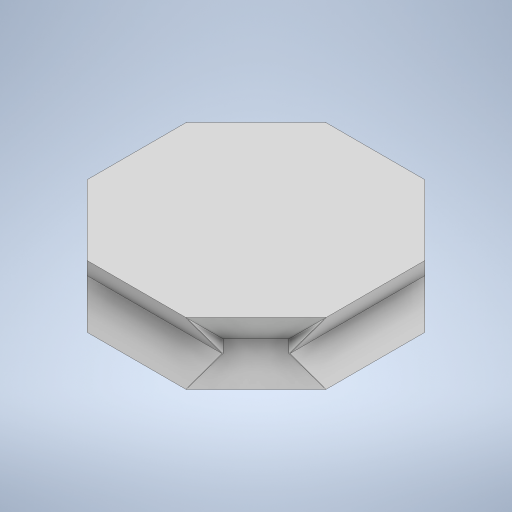
# Autodesk Inventor part: 팔각형 OV-PAM 층 한개
Saved by Autodesk Inventor 2024 (Build 280153000, 153)
## iProperties
Created: 2023-06-16
Part Number: 팔각형 OV-PAM 층 한개
Material: 일반
Document SubType Name: Modeling
Designer: jsw
Density: 1 g/cm^3
Appearance: 기본값
Mass: 146.501 g
Surface Area: 230.919 cm^2
Volume: 146.501 cm^3
Author: jsw
Autodesk Inventor part; units mm, degrees
sketch "스케치1" plane through (0, 0, 0) normal (0, 1, 0) x (-1, 0, 0)
  line L0 (-45.2922, 18.7606) -> (-18.7606, 45.2922)
  line L1 (-18.7606, 45.2922) -> (18.7606, 45.2922)
  line L2 (18.7606, 45.2922) -> (45.2922, 18.7606)
  line L3 (45.2922, 18.7606) -> (45.2922, -18.7606)
  line L4 (45.2922, -18.7606) -> (18.7606, -45.2922)
  line L5 (18.7606, -45.2922) -> (-18.7606, -45.2922)
  line L6 (-18.7606, -45.2922) -> (-45.2922, -18.7606)
  line L7 (-45.2922, -18.7606) -> (-45.2922, 18.7606)
  line L8 (-19.092, 46.0922) -> (19.092, 46.0922)
  line L9 (19.092, 46.0922) -> (46.0922, 19.092)
  line L10 (46.0922, 19.092) -> (46.0922, -19.092)
  line L11 (46.0922, -19.092) -> (19.092, -46.0922)
  line L12 (19.092, -46.0922) -> (-19.092, -46.0922)
  line L13 (-19.092, -46.0922) -> (-46.0922, -19.092)
  line L14 (-46.0922, -19.092) -> (-46.0922, 19.092)
  line L15 (-46.0922, 19.092) -> (-19.092, 46.0922)
  point P0 (0, 0)
  point P1 (0, 0)
  point P2 (0, 0)
  dimension "d2" = 0.8
  dimension "d42" = 38.184
  constraints: 32 end point, 2 coincident, 2 horizontal, 34 other
  measures "d2" distance between parallel lines of L10 L3
  measures "d42" distance of L11.end L12.end
extrude "돌출2" add sketch "스케치1" along normal blind 12 contours L0 L1 L2 L3 L4 L5 L6 L7 | L8 L9 L10 L11 L12 L13 L14 L15
ref_plane "작업 평면2" through (46.0922, 0, 19.092) normal (-0.8660254, -0.5, 0) x (0, 0, -1)
sketch "스케치3" plane through (46.0922, 0, 19.092) normal (1, 0, 0) x (0, 0, -1)
  line L0 (0, 0) -> (0, 12) projected
  line L1 (0, 12) -> (38.184, 12) projected
  line L2 (0, 0) -> (38.184, 0)
  line L3 (38.184, 0) -> (38.184, 12)
  line L4 (38.184, 12) -> (0, 12)
  line L5 (0, 12) -> (0, 0)
  line L6 (0, 12) -> (-7.3047, 12)
  line L7 (-27.0002, 12) -> (0, 12) projected
  line L8 (0, 0) -> (-7.3047, 12)
  line L9 (38.184, 12) -> (45.4887, 12)
  line L10 (45.4887, 12) -> (38.184, 0)
  point P0 (19.092, 0)
  dimension "d17" = 121.33
  dimension "d18" = 121.33
  constraints: 16 end point, 2 parallel, 2 point on line, 1 horizontal, 1 perpendicular
  measures "d17" angle of L8 L2
  measures "d18" angle of L2 L10
extrude "돌출4" cut sketch "스케치3" against normal up to surface surface through (46.0922, 0, 19.092) normal (-0.8660254, -0.5, 0)
sketch "스케치4" plane through (19.092, 0, 46.0922) normal (0.7071068, 0, 0.7071068) x (0.7071068, 0, -0.7071068)
  line L0 (0, 0) -> (0, 12) projected
  line L1 (38.184, 0) -> (38.184, 12) projected
  line L2 (0, 0) -> (38.184, 0)
  line L3 (38.184, 0) -> (38.184, 12)
  line L4 (38.184, 12) -> (0, 12)
  line L5 (0, 12) -> (0, 0)
  line L6 (38.184, 0) -> (28.386, 12) projected
  line L7 (38.184, 0) -> (28.092, 12)
  line L8 (38.184, 0) -> (0, 0) projected
  line L9 (0, 0) -> (10.092, 12)
  line L10 (38.184, 12) -> (0, 12) projected
  point P0 (19.092, 0)
  point P1 (10.092, 12)
  point P2 (19.092, 12)
  dimension "d40" = 18
  dimension "d41" = 9
  constraints: 12 end point, 2 parallel, 2 point on line, 1 horizontal, 1 midpoint, 1 perpendicular
  measures "d40" distance of L9.end L7.end
  measures "d41" distance of L7.end point (19.092, 12)
ref_plane "작업 평면3" through (19.092, 0, 46.0922) normal (0.6123724, 0.5, 0.6123724) x (0.7071068, 0, -0.7071068)
extrude "돌출5" cut sketch "스케치4" against normal up to surface contours L9 L4 L7 L2 surface through (19.092, 0, 46.0922) normal (0.6123724, 0.5, 0.6123724)
pattern_circular "원형 패턴1" count 4 over 360 about axis through (0, -10, 0) along (0, 1, 0) of "돌출4"
pattern_circular "원형 패턴2" count 4 over 360 about axis through (0, -10, 0) along (0, 1, 0) of "돌출5"
mirror "미러5" about plane through (0, 12, 0) normal (0, 1, 0) of "돌출2", "돌출5", "원형 패턴2", "돌출4", "원형 패턴1"
ref_plane "작업 평면5" through (-19.092, 12, -46.0922) normal (0, 1, 0) x (1, 0, 0)
equation "\"d41\" = 0.5 * d40"
